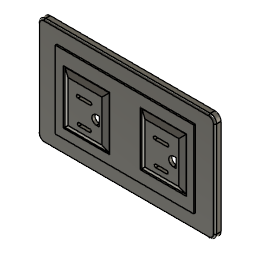
ECOSWITCH (Autodesk Fusion 360 archive; units mm, degrees)
design "Enchufe"
part number: 2026-03-28-22-37-53-552
Autodesk Fusion 360 part; units mm, degrees
sketch "Boceto1" plane through (0, 0, 0) normal (0, 1, 0) x (1, 0, 0)
  line L0 (303.7748, -214.9714) -> (196.7748, -214.9714)
  line L1 (192.7748, -218.9714) -> (192.7748, -284.9714)
  line L2 (196.7748, -284.9714) -> (303.7748, -284.9714)
  line L3 (307.7748, -280.9714) -> (307.7748, -218.9714)
  line L4 (307.7748, -214.9714) -> (192.7748, -284.9714) construction
  line L5 (192.7748, -214.9714) -> (307.7748, -284.9714) construction
  line L6 (192.7748, -280.9714) -> (192.7748, -248.4941)
  line L7 (192.7748, -248.4941) -> (217.7748, -248.4941)
  line L8 (307.7748, -250) -> (282.7748, -250)
  line L9 (282.7748, -250) -> (275.2748, -250)
  line L10 (260.2748, -232.5) -> (290.2748, -232.5)
  line L11 (290.2748, -232.5) -> (290.2748, -267.5)
  line L12 (290.2748, -267.5) -> (260.2748, -267.5)
  line L13 (260.2748, -267.5) -> (260.2748, -232.5)
  line L14 (260.2748, -232.5) -> (290.2748, -267.5) construction
  line L15 (290.2748, -232.5) -> (260.2748, -267.5) construction
  line L16 (217.7748, -248.4941) -> (225.2748, -248.4941)
  line L17 (240.2748, -230.9941) -> (210.2748, -230.9941)
  line L18 (210.2748, -230.9941) -> (210.2748, -265.9941)
  line L19 (210.2748, -265.9941) -> (240.2748, -265.9941)
  line L20 (240.2748, -265.9941) -> (240.2748, -230.9941)
  line L21 (240.2748, -230.9941) -> (210.2748, -265.9941) construction
  line L22 (210.2748, -230.9941) -> (240.2748, -265.9941) construction
  arc A0 (303.7748, -284.9714) -> (307.7748, -280.9714) centre (303.7748, -280.9714) ccw
  arc A1 (307.7748, -218.9714) -> (303.7748, -214.9714) centre (303.7748, -218.9714) ccw
  arc A2 (196.7748, -214.9714) -> (192.7748, -218.9714) centre (196.7748, -218.9714) ccw
  arc A3 (192.7748, -280.9714) -> (196.7748, -284.9714) centre (196.7748, -280.9714) ccw
  line L23 (225.2748, -265.9941) -> (225.2748, -257.4941)
  line L24 (225.2748, -230.9941) -> (225.2748, -239.4941)
  line L25 (229.4404, -254.9885) -> (221.4434, -254.9885)
  line L26 (221.4434, -256.9885) -> (229.4404, -256.9885)
  line L27 (163.1752, -254.9885) -> (212.7447, -256.9885) construction
  line L28 (212.7356, -254.9885) -> (222.7447, -256.9885) construction
  line L29 (229.0428, -239.5161) -> (222.0492, -239.5161)
  line L30 (222.0492, -241.5161) -> (229.0428, -241.5161)
  line L31 (225.2759, -239.5161) -> (225.3814, -241.5161) construction
  line L32 (225.3739, -239.5161) -> (234.3814, -241.5161) construction
  line L33 (225, -254.9885) -> (225, -241.5161)
  line L34 (225, -254.9885) -> (225, -241.5161)
  line L35 (240.2748, -248.4941) -> (232.7748, -248.4941)
  line L36 (233.5042, -245.6863) -> (235.2523, -245.6863)
  line L37 (235.2523, -245.6863) -> (235.2523, -251.6863)
  line L38 (235.2523, -251.6863) -> (233.5042, -251.6863)
  line L39 (230.5956, -245.6863) -> (235.2523, -251.6863) construction
  line L40 (235.2523, -245.6863) -> (229.9579, -251.6863) construction
  arc A4 (230.5042, -248.6975) -> (233.5042, -251.6863) centre (233.5042, -248.6863) ccw
  arc A5 (233.5042, -245.6863) -> (230.5042, -248.6975) centre (233.5042, -248.6863) ccw
  arc A6 (220.4434, -255.9921) -> (221.4434, -256.9885) centre (221.4434, -255.9885) ccw
  arc A7 (221.4434, -254.9885) -> (220.4434, -255.9921) centre (221.4434, -255.9885) ccw
  arc A8 (229.4404, -256.9885) -> (230.4404, -255.9849) centre (229.4404, -255.9885) ccw
  arc A9 (230.4404, -255.9849) -> (229.4404, -254.9885) centre (229.4404, -255.9885) ccw
  arc A10 (221.0492, -240.5205) -> (222.0492, -241.5161) centre (222.0492, -240.5161) ccw
  arc A11 (222.0492, -239.5161) -> (221.0492, -240.5205) centre (222.0492, -240.5161) ccw
  arc A12 (229.0428, -241.5161) -> (230.0427, -240.5117) centre (229.0428, -240.5161) ccw
  arc A13 (230.0427, -240.5117) -> (229.0428, -239.5161) centre (229.0428, -240.5161) ccw
  line L41 (270.7209, -257.1329) -> (278.7179, -257.1329)
  line L42 (278.7179, -255.1329) -> (270.7209, -255.1329)
  arc A14 (279.7179, -256.1293) -> (278.7179, -255.1329) centre (278.7179, -256.1329) ccw
  arc A15 (278.7179, -257.1329) -> (279.7179, -256.1293) centre (278.7179, -256.1329) ccw
  arc A16 (270.7209, -255.1329) -> (269.7209, -256.1365) centre (270.7209, -256.1329) ccw
  arc A17 (269.7209, -256.1365) -> (270.7209, -257.1329) centre (270.7209, -256.1329) ccw
  arc A18 (282.7817, -245.8307) -> (279.7817, -248.8419) centre (282.7817, -248.8307) ccw
  arc A19 (279.7817, -248.8419) -> (282.7817, -251.8307) centre (282.7817, -248.8307) ccw
  line L43 (284.5299, -251.8307) -> (282.7817, -251.8307)
  line L44 (284.5299, -245.8307) -> (284.5299, -251.8307)
  line L45 (282.7817, -245.8307) -> (284.5299, -245.8307)
  line L46 (278.3203, -239.6605) -> (271.3268, -239.6605)
  line L47 (271.3268, -241.6604) -> (278.3203, -241.6604)
  arc A20 (270.3268, -240.6649) -> (271.3268, -241.6604) centre (271.3268, -240.6604) ccw
  arc A21 (271.3268, -239.6605) -> (270.3268, -240.6649) centre (271.3268, -240.6605) ccw
  arc A22 (278.3203, -241.6604) -> (279.3203, -240.6561) centre (278.3203, -240.6604) ccw
  arc A23 (279.3203, -240.6561) -> (278.3203, -239.6605) centre (278.3203, -240.6605) ccw
  point P0 (250.2748, -249.9714)
  point P1 (275.2748, -250)
  point P2 (225.2748, -248.4941)
  point P3 (225.2748, -257.4941)
  point P4 (225.2748, -239.4941)
  point P5 (232.7748, -248.4941)
  dimension "d1" = 115
  dimension "d2" = 70
  dimension "d3" = 25
  dimension "d4" = 25
  dimension "d5" = 7.5
  dimension "d6" = 30
  dimension "d7" = 35
  dimension "d8" = 7.5
  dimension "d9" = 30
  dimension "d10" = 35
  dimension "d11" = 4
  dimension "d12" = 4
  dimension "d13" = 4
  dimension "d14" = 4
  dimension "d15" = 8.5
  dimension "d16" = 8.5
  dimension "d17" = 10
  dimension "d18" = 2
  dimension "d19" = 9
  dimension "d20" = 2
  dimension "d21" = 7.5
  dimension "d22" = 3
  dimension "d23" = 3
  dimension "d24" = 1
  dimension "d25" = 1
  dimension "d26" = 1
  dimension "d27" = 1
  dimension "d28" = 1
  dimension "d29" = 1
  dimension "d30" = 1
  dimension "d31" = 1
  dimension "d32" = 3
  dimension "d33" = 3
  dimension "d34" = 1
  dimension "d35" = 1
  dimension "d36" = 1
  dimension "d37" = 1
  dimension "d38" = 1
  dimension "d39" = 1
  dimension "d40" = 1
  dimension "d41" = 1
  constraint horizontal L0
  constraint perpendicular L0 L1
  constraint parallel L0 L2
  constraint parallel L1 L3
  constraint coincident L4 P0
  constraint coincident L5 P0
  constraint perpendicular L1 L7
  constraint perpendicular L3 L8
  constraint parallel L8 L9
  constraint horizontal L10
  constraint perpendicular L10 L11
  constraint parallel L10 L12
  constraint parallel L11 L13
  constraint coincident L14 P1
  constraint coincident L15 P1
  constraint coincident P1 L9.end
  constraint parallel L7 L16
  constraint horizontal L17
  constraint perpendicular L17 L18
  constraint parallel L17 L19
  constraint parallel L18 L20
  constraint coincident L21 P2
  constraint coincident L22 P2
  constraint coincident P2 L16.end
  constraint coincident L3 L8.start
  constraint coincident L5.end L2
  constraint coincident L5.end L3
  constraint tangent L2 A0
  constraint tangent L3 A0
  constraint coincident L4.start L0
  constraint coincident L4.start L3
  constraint tangent L0 A1
  constraint tangent L3 A1
  constraint coincident L1 L6.end
  constraint coincident L5.start L1
  constraint coincident L5.start L0
  constraint tangent L1 A2
  constraint tangent L0 A2
  constraint coincident L1.end L6
  constraint coincident L1.end L2
  constraint tangent L6 A3
  constraint tangent L2 A3
  constraint midpoint L19 L23.start
  constraint perpendicular L19 L23
  constraint midpoint L17 L24.start
  constraint perpendicular L17 L24
  constraint horizontal L25
  constraint parallel L25 L26
  constraint coincident L27 P3
  constraint coincident L28 P3
  constraint coincident P3 L23.end
  constraint horizontal L29
  constraint parallel L29 L30
  constraint coincident L31 P4
  constraint coincident L32 P4
  constraint coincident P4 L24.end
  constraint midpoint L20 L35.start
  constraint perpendicular L20 L35
  constraint horizontal L36
  constraint perpendicular L36 L37
  constraint parallel L36 L38
  constraint coincident L39 P5
  constraint coincident L40 P5
  constraint coincident P5 L35.end
  constraint coincident L40.end L38
  constraint tangent L38 A4
  constraint coincident L39.start L36
  constraint tangent L36 A5
  constraint coincident A4.start A5.end
  constraint coincident L27.end L26
  constraint tangent L26 A6
  constraint coincident L25 L33.start
  constraint coincident L28.start L25
  constraint tangent L25 A7
  constraint coincident A6.start A7.end
  constraint coincident L28.end L26
  constraint tangent L26 A8
  constraint coincident L27.start L25
  constraint tangent L25 A9
  constraint coincident A8.end A9.start
  constraint coincident L30 L33.end
  constraint coincident L31.end L30
  constraint tangent L30 A10
  constraint coincident L32.start L29
  constraint tangent L29 A11
  constraint coincident A10.start A11.end
  constraint coincident L32.end L30
  constraint tangent L30 A12
  constraint coincident L31.start L29
  constraint tangent L29 A13
  constraint coincident A12.end A13.start
  constraint horizontal L42
  constraint parallel L41 L42
  constraint horizontal L46
  constraint parallel L46 L47
  constraint horizontal L45
  constraint perpendicular L44 L45
  constraint parallel L43 L45
  constraint tangent A19 L43
  constraint tangent A18 L45
  constraint coincident A18.end A19.start
  constraint tangent L41 A17
  constraint tangent L42 A16
  constraint coincident A16.end A17.start
  constraint tangent L41 A15
  constraint tangent L42 A14
  constraint coincident A14.start A15.end
  constraint tangent L47 A20
  constraint tangent L46 A21
  constraint coincident A20.start A21.end
  constraint tangent L47 A22
  constraint tangent L46 A23
  constraint coincident A22.end A23.start
  measures "d1" distance of L1.end L5.end
  measures "d2" distance of L5.start L1.end
  measures "d3" distance of L6.end L7.end
  measures "d4" distance of L8.start L8.end
  measures "d5" distance of L8.end P1
  measures "d6" distance of L11.end L12.end
  measures "d7" distance of L10.end L11.end
  measures "d8" distance of L7.end P2
  measures "d9" distance of L18.end L19.end
  measures "d10" distance of L17.end L18.end
  measures "d11" radius of A0
  measures "d12" radius of A1
  measures "d13" radius of A2
  measures "d14" radius of A3
  measures "d15" distance of L23.start P3
  measures "d16" distance of L24.start P4
  measures "d17" distance of L27.end L28.end
  measures "d18" distance of L28.start L27.end
  measures "d19" distance of L31.end L32.end
  measures "d20" distance of L32.start L31.end
  measures "d21" distance of L35.start P5
  measures "d22" radius of A4
  measures "d23" radius of A5
  measures "d24" radius of A6
  measures "d25" radius of A7
  measures "d26" radius of A8
  measures "d27" radius of A9
  measures "d28" radius of A10
  measures "d29" radius of A11
  measures "d30" radius of A12
  measures "d31" radius of A13
  measures "d32" radius of A19
  measures "d33" radius of A18
  measures "d34" radius of A17
  measures "d35" radius of A16
  measures "d36" radius of A15
  measures "d37" radius of A14
  measures "d38" radius of A20
  measures "d39" radius of A21
  measures "d40" radius of A22
  measures "d41" radius of A23
extrude "Extruir1" add sketch "Boceto1" along normal blind 4 contours L0 L1 L2 L3 L6 A0 A1 A2 A3 makes body 1
extrude "Extruir2" add sketch "Boceto1" against normal blind 2 separate body contours L10 L11 L12 L13 makes body 2
chamfer "Chaflán1" distance 2 angle 45 2 edges at (275.2748, -2, 267.5) (260.2748, -2, 250) on bodies 2
chamfer "Chaflán2" distance 2 angle 45 2 edges at (290.2748, -2, 249) (276.2748, -2, 265.5) on bodies 2
chamfer "Chaflán3" distance 2 angle 45 2 edges at (262.2748, -2, 248) (275.2748, -2, 232.5) on bodies 2
chamfer "Chaflán4" distance 2 angle 45 2 edges at (288.2748, -2, 249) (276.2748, -2, 234.5) on bodies 2
copy_body "CopiarPegarCuerpos1" bodies 2 makes body 3
move_body "Desplazar1" bodies 3 to x (1, 0, 0) y (0, 1, 0) z (0, 0, 1) at (-49.966, 0, -1.6393)
fillet "Empalme1" radius 1 8 edges at (192.7748, 0, 249.9714) (193.9463, 0, 283.7998) (250.2748, 0, 284.9714) (306.6032, 0, 283.7998) (307.7748, 0, 249.9714) (306.6032, 0, 216.1429) (250.2748, 0, 214.9714) (193.9463, 0, 216.1429) on bodies 1
sketch "Boceto2" plane through (0, 0, 0) normal (0, -1, 0) x (1, 0, 0)
  line L0 (260.2748, 267.5) -> (290.2748, 267.5)
  line L1 (290.2748, 267.5) -> (290.2748, 232.5)
  line L2 (290.2748, 232.5) -> (260.2748, 232.5)
  line L3 (260.2748, 232.5) -> (260.2748, 267.5)
  line L4 (240.2748, 265.9941) -> (240.2748, 230.9941)
  line L5 (240.2748, 230.9941) -> (210.2748, 230.9941)
  line L6 (210.2748, 230.9941) -> (210.2748, 265.9941)
  line L7 (210.2748, 265.9941) -> (240.2748, 265.9941)
  line L8 (193.7748, 280.9714) -> (193.7748, 218.9714)
  arc A0 (193.7748, 218.9714) -> (196.7748, 215.9714) centre (196.7748, 218.9714) ccw
  line L9 (196.7748, 215.9714) -> (303.7748, 215.9714)
  arc A1 (303.7748, 215.9714) -> (306.7748, 218.9714) centre (303.7748, 218.9714) ccw
  line L10 (306.7748, 218.9714) -> (306.7748, 280.9714)
  arc A2 (306.7748, 280.9714) -> (303.7748, 283.9714) centre (303.7748, 280.9714) ccw
  line L11 (303.7748, 283.9714) -> (196.7748, 283.9714)
  arc A3 (196.7748, 283.9714) -> (193.7748, 280.9714) centre (196.7748, 280.9714) ccw
  line L12 (205, 275) -> (295, 275)
  line L13 (295, 275) -> (295, 225)
  line L14 (295, 225) -> (205, 225)
  line L15 (205, 225) -> (205, 275)
  line L16 (205, 275) -> (295, 225) construction
  line L17 (295, 275) -> (205, 225) construction
  point P0 (250, 250)
  constraint horizontal L12
  constraint perpendicular L12 L13
  constraint parallel L12 L14
  constraint parallel L13 L15
  constraint coincident L16 P0
  constraint coincident L17 P0
extrude "Extruir6" add sketch "Boceto2" along normal blind 1 contours L12 L13 L14 L15 bodies 1 3 2

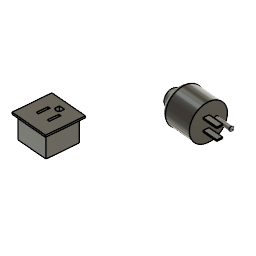
design "Nema Hembra y Macho"
part number: 2026-03-30-18-51-31-380
Autodesk Fusion 360 part; units mm, degrees
sketch "Boceto1" plane through (0, 0, 0) normal (0, 0, 1) x (1, 0, 0)
  circle A0 centre (75, 55) radius 20
  dimension "d1" = 40
  measures "d1" diameter of A0
extrude "Extruir1" add sketch "Boceto1" along normal blind 35 makes body 1
fillet "Empalme1" radius 5 1 faces at (63.8127, 57.6911, 0) on bodies 1
sketch "Boceto2" plane through (0, 0, 35) normal (0, 0, 1) x (-1, 0, 0)
  circle A0 centre (-75, -55) radius 20
  circle A1 centre (-75, -63.1) radius 2.4
  line L0 (-75, -75) -> (-75, -63.1)
  line L1 (-80.7445, -55.7276) -> (-82.2445, -55.7276)
  line L2 (-82.2445, -55.7276) -> (-82.2445, -49.4276)
  line L3 (-82.2445, -49.4276) -> (-80.7445, -49.4276)
  line L4 (-80.7445, -49.4276) -> (-80.7445, -55.7276)
  line L5 (-80.7445, -55.7276) -> (-82.2445, -49.4276) construction
  line L6 (-82.2445, -55.7276) -> (-80.7445, -49.4276) construction
  line L7 (-81.4945, -52.5776) -> (-68.7945, -52.5776)
  line L8 (-68.0445, -55.7276) -> (-69.5445, -55.7276)
  line L9 (-69.5445, -55.7276) -> (-69.5445, -49.4276)
  line L10 (-69.5445, -49.4276) -> (-68.0445, -49.4276)
  line L11 (-68.0445, -49.4276) -> (-68.0445, -55.7276)
  line L12 (-68.0445, -55.7276) -> (-69.5445, -49.4276) construction
  line L13 (-69.5445, -55.7276) -> (-68.0445, -49.4276) construction
  line L14 (-75, -35) -> (-75, -56.7166)
  point P0 (-81.4945, -52.5776)
  point P1 (-68.7945, -52.5776)
  dimension "d6" = 4.8
  dimension "d7" = 11.9
  dimension "d8" = 1.5
  dimension "d9" = 6.3
  dimension "d10" = 12.7
  dimension "d11" = 1.5
  dimension "d12" = 6.3
  constraint coincident A0 L0.start
  constraint vertical L0
  constraint coincident A1.centre L0.end
  constraint horizontal L1
  constraint perpendicular L1 L2
  constraint parallel L1 L3
  constraint parallel L2 L4
  constraint coincident L5 P0
  constraint coincident L6 P0
  constraint coincident P0 L7.start
  constraint perpendicular L4 L7
  constraint horizontal L8
  constraint perpendicular L8 L9
  constraint parallel L8 L10
  constraint parallel L9 L11
  constraint coincident L12 P1
  constraint coincident L13 P1
  constraint coincident P1 L7.end
  constraint coincident A0 L14.start
  constraint vertical L14
  measures "d6" diameter of A1
  measures "d7" distance of L0.start A1.centre
  measures "d8" distance of L2.end L3.end
  measures "d9" distance of L1.end L2.end
  measures "d10" distance of P0 P1
  measures "d11" distance of L9.end L10.end
  measures "d12" distance of L8.end L9.end
extrude "Extruir2" add sketch "Boceto2" along normal blind 17 contours L1 L2 L3 L4 | L8 L9 L10 L11 bodies 1
extrude "Extruir3" add sketch "Boceto2" along normal blind 21 contours A1 bodies 1
fillet "Empalme2" radius 2 1 faces at (74.5012, 62.0029, 56) on bodies 1
sketch "Boceto3" plane through (0, 0, 0) normal (0, 0, -1) x (1, 0, 0)
  circle A0 centre (75, -55) radius 15
  circle A1 centre (75, -55) radius 9
  dimension "d19" = 18
  constraint concentric A0 A1
  measures "d19" diameter of A1
extrude "Extruir4" add sketch "Boceto3" along normal blind 10 contours A1 bodies 1
sketch "Boceto10" plane through (0, 0, 0) normal (0, 0, 1) x (1, 0, 0)
  line L0 (95.7817, -50.9127) -> (53.7817, -50.9127)
  line L1 (53.7817, -50.9127) -> (53.7817, -8.9127)
  line L2 (53.7817, -8.9127) -> (95.7817, -8.9127)
  line L3 (95.7817, -8.9127) -> (95.7817, -50.9127)
  line L4 (95.7817, -50.9127) -> (53.7817, -8.9127) construction
  line L5 (53.7817, -50.9127) -> (95.7817, -8.9127) construction
  line L6 (74.7817, -8.9127) -> (74.7817, -29.9127)
  line L7 (95.7817, -29.9127) -> (74.7817, -29.9127)
  line L8 (85.2817, -29.9127) -> (85.2817, -8.9127)
  line L9 (85.2817, -29.9127) -> (65, -29.9127)
  line L10 (69.201, -35.9127) -> (66.701, -35.9127)
  line L11 (66.701, -35.9127) -> (66.701, -23.9127)
  line L12 (66.701, -23.9127) -> (69.201, -23.9127)
  line L13 (69.201, -23.9127) -> (69.201, -35.9127)
  line L14 (69.201, -35.9127) -> (66.701, -23.9127) construction
  line L15 (66.701, -35.9127) -> (69.201, -23.9127) construction
  line L16 (80.3485, -23.9127) -> (82.8485, -23.9127)
  line L17 (82.8485, -23.9127) -> (82.8485, -35.9127)
  line L18 (82.8485, -35.9127) -> (80.3485, -35.9127)
  line L19 (80.3485, -35.9127) -> (80.3485, -23.9127)
  line L20 (80.3485, -23.9127) -> (82.8485, -35.9127) construction
  line L21 (82.8485, -23.9127) -> (80.3485, -35.9127) construction
  line L22 (77.7817, -43.6849) -> (71.7817, -43.6849)
  line L23 (71.7817, -43.6849) -> (71.7817, -39.6849)
  line L24 (73.7817, -37.6849) -> (75.7817, -37.6849)
  line L25 (77.7817, -39.6849) -> (77.7817, -43.6849)
  line L26 (77.7817, -43.6849) -> (71.7817, -37.6849) construction
  line L27 (71.7817, -43.6849) -> (77.7817, -37.6849) construction
  arc A0 (73.7817, -37.6849) -> (71.7817, -39.6849) centre (73.7817, -39.6849) ccw
  arc A1 (77.7817, -39.6849) -> (75.7817, -37.6849) centre (75.7817, -39.6849) ccw
  line L28 (57.3512, -47.3433) -> (92.3512, -47.3433)
  line L29 (92.3512, -47.3433) -> (92.3512, -12.3433)
  line L30 (92.3512, -12.3433) -> (57.3512, -12.3433)
  line L31 (57.3512, -12.3433) -> (57.3512, -47.3433)
  point P0 (74.7817, -29.9127)
  point P1 (67.951, -29.9127)
  point P2 (81.5985, -29.9127)
  point P3 (74.7817, -40.6849)
  dimension "d56" = 42
  dimension "d57" = 42
  dimension "d58" = 2.5
  dimension "d59" = 12
  dimension "d60" = 2.5
  dimension "d61" = 12
  dimension "d62" = 6
  dimension "d63" = 6
  dimension "d64" = 2
  dimension "d65" = 2
  dimension "d68" = 35
  dimension "d69" = 35
  constraint horizontal L0
  constraint perpendicular L0 L1
  constraint parallel L0 L2
  constraint parallel L1 L3
  constraint coincident L4 P0
  constraint coincident L5 P0
  constraint midpoint L2 L6.start
  constraint coincident P0 L6.end
  constraint midpoint L3 L7.start
  constraint midpoint L7 L8.start
  constraint coincident L2 L8.end
  constraint perpendicular L2 L8
  constraint perpendicular L6 L9
  constraint horizontal L10
  constraint perpendicular L10 L11
  constraint parallel L10 L12
  constraint parallel L11 L13
  constraint coincident L14 P1
  constraint coincident L15 P1
  constraint coincident L9 P1
  constraint horizontal L16
  constraint perpendicular L16 L17
  constraint parallel L16 L18
  constraint parallel L17 L19
  constraint coincident L20 P2
  constraint coincident L21 P2
  constraint coincident L7 P2
  constraint horizontal L22
  constraint perpendicular L22 L23
  constraint parallel L22 L24
  constraint parallel L23 L25
  constraint coincident L26 P3
  constraint coincident L27 P3
  constraint coincident L26.end L23
  constraint coincident L26.end L24
  constraint tangent L23 A0
  constraint tangent L24 A0
  constraint coincident L27.end L24
  constraint coincident L27.end L25
  constraint tangent L24 A1
  constraint tangent L25 A1
  constraint horizontal L28
  constraint vertical L29
  constraint horizontal L30
  constraint vertical L31
  constraint coincident L5 L28.start
  measures "d56" distance of L1.end L2.end
  measures "d57" distance of L0.end L1.end
  measures "d58" distance of L11.end L12.end
  measures "d59" distance of L10.end L11.end
  measures "d60" distance of L17.end L18.end
  measures "d61" distance of L16.end L17.end
  measures "d62" distance of L26.end L27.end
  measures "d63" distance of L22.end L26.end
  measures "d64" radius of A0
  measures "d65" radius of A1
  measures "d68" distance of L28.start L28.end
  measures "d69" distance of L28.start L30.end
extrude "Extruir11" add sketch "Boceto10" along normal blind 2 separate body contours L0 L1 L2 L3 L6 L7 L28 L29 L30 L31 | L2 L3 L7 L8 L29 L30 | L6 L7 L9 L17 L18 L19 L28 L29 L30 L31 | L7 L8 L29 L30 | L2 L6 L8 L30 | L6 L7 L8 L9 L16 L17 L19 L30 makes body 2
extrude "Extruir12" add sketch "Boceto10" against normal blind 25 separate body contours L6 L7 L9 L17 L18 L19 L28 L29 L30 L31 | L7 L8 L29 L30 | L6 L7 L8 L9 L16 L17 L19 L30 makes body 3
extrude "Extruir13" add sketch "Boceto10" against normal blind 31 contours L7 L9 L17 L18 L19 | L7 L9 L16 L17 L19 | L9 L10 L11 L13 | L9 L11 L12 L13 | L22 L23 L24 L25 A0 A1 bodies 2 3
extrude "Extruir14" cut 3 faces at (68.3677, -27.9127, 0) (81.1819, -27.9127, 0) (75.7817, -42.3516, 0) along direction (0, 0, -1) blind 19 on bodies 2 bodies 2
move_body "Desplazar1" bodies 2 to x (1, 0, 0) y (0, -1, 0) z (0, 0, -1) at (0, -101.8254, -62)
move_body "Desplazar2" bodies 2 to x (1, 0, 0) y (0, 1, 0) z (0, 0, 1) at (0, 126, 0)
move_body "Desplazar3" bodies 2 to x (1, 0, 0) y (0, 1, 0) z (0, 0, 1) at (0, 0, -5)
move_body "Desplazar4" bodies 1 to x (0, 0, -1) y (0.087156, 0.996195, 0) z (0.996195, -0.087156, 0) at (191.9115, -60.7384, 45)
move_body "Desplazar5" bodies 2 to x (0.996195, -0.087156, 0) y (0.087156, 0.996195, 0) z (0, 0, 1) at (71.5064, 56.1587, 0)
move_body "Desplazar6" bodies 2 to x (1, 0, 0) y (0, 1, 0) z (0, 0, 1) at (0, 5, 0)
move_body "Desplazar7" bodies 2 to x (1, 0, 0) y (0, 1, 0) z (0, 0, 1) at (0, 0, 30)
move_body "Desplazar8" bodies 2 to x (-1, 0, 0) y (0, 1, 0) z (0, 0, -1) at (255.9345, 0, -78)
move_body "Desplazar9" bodies 2 to x (1, 0, 0) y (0, 1, 0) z (0, 0, 1) at (60, 0, 40)
move_body "Desplazar10" bodies 2 to x (1, 0, 0) y (0, 1, 0) z (0, 0, 1) at (-10, 0, 0)
move_body "Desplazar11" bodies 2 to x (1, 0, 0) y (0, 1, 0) z (0, 0, 1) at (-1, 0, 0)
move_body "Desplazar12" bodies 2 to x (1, 0, 0) y (0, 1, 0) z (0, 0, 1) at (0, -2, 0)
move_body "Desplazar13" bodies 2 to x (0.984808, -0.173648, 0) y (0.173648, 0.984808, 0) z (0, 0, 1) at (-12.5496, 24.1016, 0)
move_body "Desplazar14" bodies 2 to x (1, 0, 0) y (0, 1, 0) z (0, 0, 1) at (-5, 0, 0)
move_body "Desplazar15" bodies 2 to x (1, 0, 0) y (0, 1, 0) z (0, 0, 1) at (0, 0, -10)
move_body "Desplazar16" bodies 2 to x (1, 0, 0) y (0, 1, 0) z (0, 0, 1) at (0, 5, 0)
move_body "Desplazar17" bodies 2 to x (1, 0, 0) y (0, 1, 0) z (0, 0, 1) at (-1, 0, 0)
move_body "Desplazar18" bodies 2 to x (1, 0, 0) y (0, 1, 0) z (0, 0, 1) at (-2, 0, 0)
move_body "Desplazar19" bodies 2 to x (1, 0, 0) y (0, 1, 0) z (0, 0, 1) at (3, 0, 0)
move_body "Desplazar20" bodies 2 to x (1, 0, 0) y (0, 1, 0) z (0, 0, 1) at (1, 0, 0)
move_body "Desplazar21" bodies 2 to x (1, 0, 0) y (0, 1, 0) z (0, 0, 1) at (0, -220, 0)

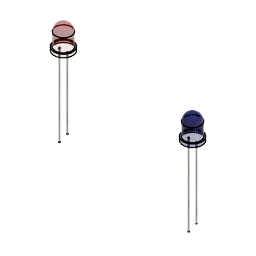
design "Led's Rojo y azul"
part number: 2026-03-28-21-06-32-198
Autodesk Fusion 360 part; units mm, degrees
sketch "Boceto1" plane through (0, 0, 0) normal (0, 0, 1) x (1, 0, 0)
  circle A0 centre (52.0206, 41.8833) radius 2.95
  circle A1 centre (-7, -7) radius 2.95
  circle A2 centre (-7, -7) radius 2.5
  line L0 (-9.95, -7.0073) -> (-9.5, -7.0073)
  dimension "d1" = 5.9
  dimension "d2" = 5.9
  dimension "d3" = 5
  dimension "d4" = 0.45
  constraint concentric A1 A2
  constraint coincident A1 L0.start
  constraint coincident A2 L0.end
  constraint horizontal L0
  measures "d1" diameter of A0
  measures "d2" diameter of A1
  measures "d3" diameter of A2
  measures "d4" distance of L0.start L0.end
extrude "Extruir1" add sketch "Boceto1" along normal blind 7.6 contours A2 makes body 1
extrude "Extruir2" add sketch "Boceto1" along normal blind 1 contours A1 bodies 1
fillet "Empalme1" radius 2.5 1 faces at (-6.1414, -6.4146, 7.6) on bodies 1
sketch "Boceto2" plane through (0, 0, 0) normal (0, 0, -1) x (1, 0, 0)
  circle A0 centre (-7, 7) radius 2.95
  line L0 (-9.5, 7) -> (-8.23, 7)
  circle A1 centre (-8.23, 7) radius 0.25
  line L1 (-4.5, 7) -> (-5.77, 7)
  circle A2 centre (-5.77, 7) radius 0.25
  dimension "d11" = 1.27
  dimension "d12" = 0.5
  dimension "d13" = 1.27
  dimension "d14" = 0.5
  constraint horizontal L0
  constraint coincident L0.end A1.centre
  constraint horizontal L1
  constraint coincident L1.end A2.centre
  measures "d11" distance of L0.start L0.end
  measures "d12" diameter of A1
  measures "d13" distance of L1.start L1.end
  measures "d14" diameter of A2
extrude "Extruir3" add sketch "Boceto2" along normal blind 25.4 contours A1 bodies 1
extrude "Extruir4" add sketch "Boceto2" along normal blind 22 contours A2 bodies 1
copy_body "CopiarPegarCuerpos1" bodies 1 makes body 2
move_body "Desplazar1" bodies 2 to x (1, 0, 0) y (0, 1, 0) z (0, 0, 1) at (12.4799, -0.1156, 0)
move_body "Desplazar2" bodies 1 to x (1, 0, 0) y (0, 1, 0) z (0, 0, 1) at (-20, 0, 0)
move_body "Desplazar3" bodies 2 to x (1, 0, 0) y (0, 1, 0) z (0, 0, 1) at (5, 0, 0)
move_body "Desplazar4" bodies 2 to x (1, 0, 0) y (0, 1, 0) z (0, 0, 1) at (5, 0, 0)
move_body "Desplazar5" bodies 2 to x (1, 0, 0) y (0, 1, 0) z (0, 0, 1) at (0, 0, -5)
move_body "Desplazar6" bodies 2 to x (1, 0, 0) y (0, 1, 0) z (0, 0, 1) at (-3, 0, 0)
move_body "Desplazar7" bodies 1 to x (1, 0, 0) y (0, 1, 0) z (0, 0, 1) at (0, 1, 0)
move_body "Desplazar8" bodies 1 to x (1, 0, 0) y (0, 1, 0) z (0, 0, 1) at (0, 1, 0)
move_body "Desplazar9" bodies 1 to x (1, 0, 0) y (0, 1, 0) z (0, 0, 1) at (-1, 0, 0)
move_body "Desplazar10" bodies 1 to x (1, 0, 0) y (0, 1, 0) z (0, 0, 1) at (-1, 0, 0)
move_body "Desplazar11" bodies 1 to x (1, 0, 0) y (0, 1, 0) z (0, 0, 1) at (-1, 0, 0)
move_body "Desplazar12" bodies 1 to x (1, 0, 0) y (0, 1, 0) z (0, 0, 1) at (0, 0, -10)
move_body "Desplazar13" bodies 2 to x (1, 0, 0) y (0, 1, 0) z (0, 0, 1) at (0, 0, -7)
named bodies: "Rojo", "Azul"

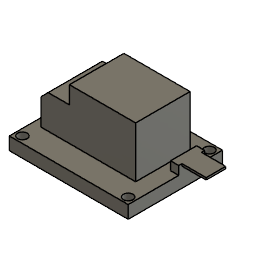
design "rele"
part number: 2026-03-25-11-49-12-979
Autodesk Fusion 360 part; units mm, degrees
sketch "Boceto1" plane through (0, 0, 0) normal (0, 1, 0) x (1, 0, 0)
  line L0 (16.7, -13.25) -> (-16.7, -13.25)
  line L1 (-16.7, -13.25) -> (-16.7, 13.25)
  line L2 (-16.7, 13.25) -> (16.7, 13.25)
  line L3 (16.7, 13.25) -> (16.7, -13.25)
  line L4 (16.7, -13.25) -> (-16.7, 13.25) construction
  line L5 (-16.7, -13.25) -> (16.7, 13.25) construction
  line L6 (-14.4, 8.65) -> (12.2, 8.65)
  line L7 (12.2, 8.65) -> (12.2, -6.65)
  line L8 (12.2, -6.65) -> (-14.4, -6.65)
  line L9 (-14.4, -6.65) -> (-14.4, 8.65)
  line L10 (-6.4, 8.65) -> (-6.4, -6.65)
  circle A0 centre (-14.85, 11.4) radius 1.35
  circle A1 centre (14.85, 11.4) radius 1.35
  circle A2 centre (14.85, -11.4) radius 1.35
  circle A3 centre (-14.85, -11.4) radius 1.35
  line L11 (14.4, 8.25) -> (16.7, 8.25)
  line L12 (16.7, 8.25) -> (16.7, 0.95)
  line L13 (16.7, 0.95) -> (14.4, 0.95)
  line L14 (14.4, 0.95) -> (14.4, 8.25)
  dimension "d1" = 33.4
  dimension "d2" = 26.5
  dimension "d3" = 26.6
  dimension "d4" = 15.3
  dimension "d5" = 4.6
  dimension "d6" = 4.5
  dimension "d8" = 8
  dimension "d16" = 2.7
  dimension "d17" = 1.85
  dimension "d18" = 1.85
  dimension "d19" = 1.85
  dimension "d20" = 1.85
  dimension "d21" = 5
  dimension "d22" = 2.3
  dimension "d23" = 7.3
  constraint horizontal L0
  constraint perpendicular L0 L1
  constraint parallel L0 L2
  constraint parallel L1 L3
  constraint coincident L4 origin
  constraint coincident L5 origin
  constraint horizontal L6
  constraint vertical L7
  constraint horizontal L8
  constraint vertical L9
  constraint coincident L6 L10.start
  constraint coincident L8 L10.end
  constraint perpendicular L8 L10
  constraint equal A0 A1
  constraint equal A1 A2
  constraint equal A2 A3
  constraint horizontal A0.centre A1.centre
  constraint vertical A0.centre A3.centre
  constraint horizontal A2.centre A3.centre
  constraint vertical A1.centre A2.centre
  constraint horizontal L11
  constraint vertical L12
  constraint horizontal L13
  constraint vertical L14
  constraint collinear L3 L12
  measures "d1" distance of L1.end L2.end
  measures "d2" distance of L0.start L2.end
  measures "d3" distance of L7 L9
  measures "d4" distance of L6.end L7.end
  measures "d5" distance of L2 L6
  measures "d6" distance of L3 L7
  measures "d8" distance of L9 L10
  measures "d16" diameter of A0
  measures "d17" distance of L2 A0.centre
  measures "d18" distance of L1 A0.centre
  measures "d19" distance of L3 A1.centre
  measures "d20" distance of L0 A2.centre
  measures "d21" distance of L2 L11
  measures "d22" distance of L12 L14
  measures "d23" distance of L11.start L13.end
extrude "Extruir1" add sketch "Boceto1" along normal blind 3.6 contours L0 L1 L2 L3 L11 L13 L14 | L3 L11 L12 L13 L14 | L6 L8 L9 L10 | L6 L7 L8 L10
extrude "Extruir2" add sketch "Boceto1" along normal blind 17.9 contours L6 L7 L8 L10
extrude "Extruir3" add sketch "Boceto1" along normal blind 13 contours L6 L8 L9 L10
chamfer "Chaflán1" distance 2 angle 45 1 edges at (-14.4, 13, -1)
extrude "Extruir4" add sketch "Boceto1" along normal blind 6 contours L3 L11 L12 L13 L14
sketch "Boceto2" plane through (16.7, 0, 0) normal (1, 0, 0) x (0, 0, -1)
  line L0 (0.95, 3.6) -> (-13.25, 3.6)
  line L1 (-13.25, 3.6) -> (-13.25, 0)
  line L2 (-13.25, 0) -> (13.25, 0)
  line L3 (13.25, 0) -> (13.25, 3.6)
  line L4 (13.25, 3.6) -> (8.25, 3.6)
  line L5 (8.25, 3.6) -> (8.25, 6)
  line L6 (8.25, 6) -> (0.95, 6)
  line L7 (0.95, 6) -> (0.95, 3.6)
  line L8 (1.85, 6) -> (7.35, 6)
  line L9 (7.35, 6) -> (7.35, 5.4)
  line L10 (7.35, 5.4) -> (1.85, 5.4)
  line L11 (1.85, 5.4) -> (1.85, 6)
  point P0 (4.6, 6)
  point P1 (4.6, 6)
  dimension "d26" = 0.6
  dimension "d27" = 5.5
  constraint horizontal L8
  constraint vertical L9
  constraint horizontal L10
  constraint vertical L11
  constraint midpoint L8 P1
  constraint midpoint L6 P1
  constraint vertical P1 P0
  constraint coincident P1 P0
  measures "d26" distance of L8.end L9.end
  measures "d27" distance of L8.start L8.end
extrude "Extruir5" add sketch "Boceto2" along normal blind 6.8 contours L6 L8 L9 L10 L11
equation "d9 = 1.2 mm + 2.4 mm"
equation "d11 = 16.7 mm + 1.2 mm"
equation "d17 = 0.5 mm + ( ( 2.7 / 2 ) * 1 mm )"
equation "d18 = 0.5 mm + ( ( 2.7 / 2 ) * 1 mm )"
equation "d19 = 0.5 mm + ( ( 2.7 / 2 ) * 1 mm )"
equation "d20 = 0.5 mm + ( ( 2.7 / 2 ) * 1 mm )"
